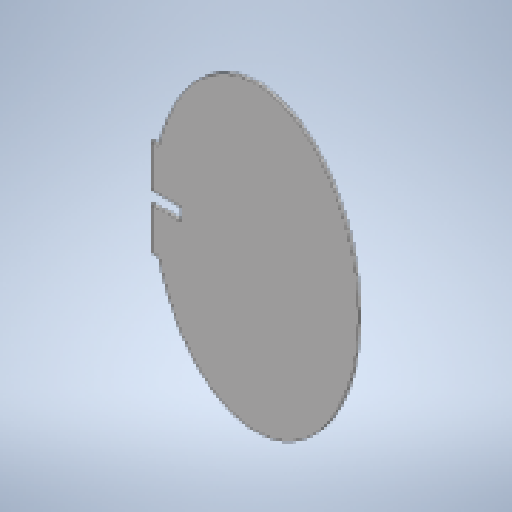
# Autodesk Inventor part: лицо
Saved by Autodesk Inventor 2023 (Build 270158000, 158)
## iProperties
Created: 2025-02-03
Part Number: лицо
Material: Типовые
Document SubType Name: Modeling
Designer: baranovaem
Density: 1 g/cm^3
Appearance: По умолчанию
Author: baranovaem
Autodesk Inventor part; units mm, degrees
ref_plane "YZ Plane" through (0, 0, 0) normal (1, 0, 0) x (0, 1, 0)
ref_plane "XZ Plane" through (0, 0, 0) normal (0, 1, 0) x (-1, 0, 0)
ref_plane "XY Plane" through (0, 0, 0) normal (0, 0, 1) x (1, 0, 0)
sketch "Эскиз1" plane through (0, 0, 0) normal (0, 0, 1) x (1, 0, 0)
  line L0 (-3.9038, 80.0048) -> (0.0962, 79.9999)
  line L1 (0.012, 10) -> (-3.988, 10.0048)
  line L2 (-3.988, 10.0048) -> (-3.9038, 80.0048)
  line L3 (-0.0962, -79.9999) -> (-4.0962, -79.9951)
  line L4 (-4.0962, -79.9951) -> (-4.0871, -72.4461)
  line L5 (-4.0616, -51.1855) -> (-4.012, -9.9952)
  line L6 (-4.012, -9.9952) -> (-0.012, -10)
  ellipse E0 centre (225, 0) end of major axis (225, -300) minor radius 225 (8.1475, -79.9999) -> (8.1475, 79.9999) ccw
  line L7 (0.0962, 79.9999) -> (8.1475, 79.9999)
  line L8 (8.1475, -79.9999) -> (-0.0962, -79.9999)
  line L9 (-4.0616, -51.1855) -> (-4.0871, -72.4461)
  line L10 (22, 79.9999) -> (22, 79.9736)
  line L11 (0.012, 10) -> (46.012, 10)
  line L12 (46.012, 10) -> (46.012, -10)
  line L13 (46.012, -10) -> (-0.012, -10)
  point P0 (0, 0)
  dimension "d0" = 300
  dimension "d1" = 225
  constraints: 28 end point, 4 perpendicular, 2 horizontal, 1 point on line, 22 other
extrude "Выдавливание1" add sketch "Эскиз1" along normal mid plane 4
sketch "Эскиз2" plane through (0, 0, 2) normal (0, 0, 1) x (1, 0, 0)
  line L0 (330, 177.5) -> (120, 177.5)
  line L1 (120, 177.5) -> (120, -177.5)
  line L2 (120, -177.5) -> (330, -177.5)
  line L3 (330, -177.5) -> (330, 177.5)
  ellipse E0 centre (225, 0) end of major axis (225, -300) minor radius 225 (8.1475, -79.9999) -> (8.1475, 79.9999) ccw projected
  line L4 (330, 177.5) -> (120, -177.5) construction
  line L5 (330, -177.5) -> (120, 177.5) construction
  point P0 (225, 0)
  dimension "d6" = 210
  dimension "d7" = 355
  constraints: 12 end point, 2 parallel, 1 coincident, 1 horizontal, 1 midpoint, 1 perpendicular, 1 other
  measures "d6" distance of L2.end L1.end
  measures "d7" distance of L1.end L0.end
